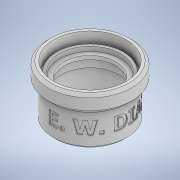
# Autodesk Inventor part: Union_Camara_E_Diaz
Saved by Autodesk Inventor 2021 (Build 250183000, 183)
## iProperties
Created: 2021-02-05
Part Number: Union_Camara_E_Diaz
Material: Generic
Document SubType Name: Modeling
Designer: jorge
Density: 1 g/cm^3
Appearance: Default
Author: jorge
Autodesk Inventor part; units mm, degrees
note: some values were not read from the file. Chosen so that the rebuilt part matches the saved one: direction of "Emboss1".
ref_plane "YZ Plane" through (0, 0, 0) normal (1, 0, 0) x (0, 1, 0)
ref_plane "XZ Plane" through (0, 0, 0) normal (0, 1, 0) x (-1, 0, 0)
ref_plane "XY Plane" through (0, 0, 0) normal (0, 0, 1) x (1, 0, 0)
sketch "Sketch1" plane through (0, 0, 0) normal (0, 1, 0) x (-1, 0, 0)
  circle A0 centre (0, 0) radius 16.8
  circle A1 centre (0, 0) radius 19.8
  dimension "d0" = 33.6
  dimension "d1" = 3
  constraints: 2 centre point, 1 coincident
  measures "d0" diameter of A0
  measures "d1" radial gap between concentric circles of A0 A1
extrude "Extrusion1" add sketch "Sketch1" along normal blind 20
sketch "Sketch2" plane through (0, 20, 0) normal (0, 1, 0) x (1, 0, 0)
  circle A0 centre (0, 0) radius 19.5
  circle A1 centre (0, 0) radius 22.5
  dimension "d4" = 39
  dimension "d5" = 3
  constraints: 2 centre point, 1 coincident
  measures "d4" diameter of A0
  measures "d5" radial gap between concentric circles of A0 A1
extrude "Extrusion2" add sketch "Sketch2" along normal blind 7.5
chamfer "Chamfer1" distance 2.7 angle 45 1 edges at (19.8, 20, 0)
sketch "Sketch3" plane through (0, 20, 0) normal (0, 1, 0) x (1, 0, 0)
  circle A0 centre (0, 0) radius 14
  circle A1 centre (0, 0) radius 16.8
  circle A2 centre (0, 0) radius 16.8 projected
  dimension "d11" = 28
  constraints: 2 centre point, 2 coincident, 1 concentric
  measures "d11" diameter of A0
extrude "Extrusion3" add sketch "Sketch3" against normal blind 2
sketch "Sketch4" plane through (0, 18, 0) normal (0, -1, 0) x (1, 0, 0)
  circle A0 centre (0, 0) radius 15.7
  circle A1 centre (0, 0) radius 16.8
  circle A2 centre (0, 0) radius 16.8 projected
  dimension "d14" = 31.4
  constraints: 2 centre point, 2 coincident, 1 concentric
  measures "d14" diameter of A0
extrude "Extrusion4" add sketch "Sketch4" along normal blind 5
sketch "Sketch5" plane through (0, 27.5, 0) normal (0, 1, 0) x (1, 0, 0)
  circle A0 centre (0, 0) radius 18
  circle A1 centre (0, 0) radius 19.5 projected
  circle A2 centre (0, 0) radius 16.5
  dimension "d17" = 1.5
  dimension "d18" = 3
  constraints: 2 centre point, 2 coincident
  measures "d17" radial gap between concentric circles of A1 A0
  measures "d18" radial gap between concentric circles of A2 A1
extrude "Extrusion5" add sketch "Sketch5" against normal up to surface (7.5 mm away) contours A0
chamfer "Chamfer2" distance 1.5 angle 45 1 edges at (-22.5, 27.5, 0)
sketch "Sketch6" plane through (0, 27.5, 0) normal (0, 1, 0) x (1, 0, 0)
  circle A0 centre (0, 0) radius 18
  circle A1 centre (0, 0) radius 18 projected
  constraints: 1 centre point, 1 coincident, 1 concentric
extrude "Extrusion6" cut sketch "Sketch6" against normal blind 5
chamfer "Chamfer3" distance 1.5 angle 45 1 edges at (19.8, 0, 0)
sketch "Sketch7" plane through (0, 0, 0) normal (1, 0, 0) x (0, 1, 0)
  line L0 (13.6432, 34.118) -> (13.6432, -36.6439) construction
  line L1 (13.6432, -36.6439) -> (5.5986, -36.6439) construction
  line L2 (5.5986, -36.6439) -> (5.5986, 34.118) construction
  line L3 (5.5986, 34.118) -> (13.6432, 34.118) construction
  line L4 (6.6432, 33.3919) -> (13.6432, 33.3919)
  line L5 (13.6432, 33.3919) -> (13.6432, 28.6609)
  line L6 (13.6432, 28.6609) -> (12.3101, 28.6609)
  line L7 (12.3101, 28.6609) -> (12.3101, 31.6447)
  line L8 (12.3101, 31.6447) -> (11.0791, 31.6447)
  line L9 (11.0791, 31.6447) -> (11.0791, 28.8935)
  line L10 (11.0791, 28.8935) -> (9.7461, 28.8935)
  line L11 (9.7461, 28.8935) -> (9.7461, 31.6447)
  line L12 (9.7461, 31.6447) -> (7.9762, 31.6447)
  line L13 (7.9762, 31.6447) -> (7.9762, 28.6609)
  line L14 (7.9762, 28.6609) -> (6.6432, 28.6609)
  line L15 (6.6432, 28.6609) -> (6.6432, 33.3919)
  line L16 (6.6432, 25.8643) -> (6.6432, 27.5264)
  line L17 (6.6432, 27.5264) -> (8.4924, 27.5264)
  line L18 (8.4924, 27.5264) -> (8.4924, 25.8643)
  line L19 (8.4924, 25.8643) -> (6.6432, 25.8643)
  line L20 (13.6432, 12.6188) -> (6.6432, 14.3886)
  line L21 (6.6432, 14.3886) -> (6.6432, 16.3173)
  line L22 (6.6432, 16.3173) -> (10.9714, 17.4405)
  line L23 (10.9714, 17.4405) -> (6.6432, 18.524)
  line L24 (6.6432, 18.524) -> (6.6432, 20.4583)
  line L25 (6.6432, 20.4583) -> (13.6432, 22.2282)
  line L26 (13.6432, 22.2282) -> (13.6432, 20.4016)
  line L27 (13.6432, 20.4016) -> (8.9576, 19.4373)
  line L28 (8.9576, 19.4373) -> (13.6432, 18.2687)
  line L29 (13.6432, 18.2687) -> (13.6432, 16.5216)
  line L30 (13.6432, 16.5216) -> (8.9519, 15.4097)
  line L31 (8.9519, 15.4097) -> (13.6432, 14.4)
  line L32 (13.6432, 14.4) -> (13.6432, 12.6188)
  line L33 (6.6432, 10.1455) -> (6.6432, 11.8076)
  line L34 (6.6432, 11.8076) -> (8.4924, 11.8076)
  line L35 (8.4924, 11.8076) -> (8.4924, 10.1455)
  line L36 (8.4924, 10.1455) -> (6.6432, 10.1455)
  spline S0 degree 2 poles (10.1375, -0.3204) (9.1561, -0.3204) (7.6132, 0.5361) (7.1991, 1.1885) knots 0 0 0 1 2 2 2
  spline S1 degree 2 poles (7.1991, 1.1885) (6.8474, 1.7331) (6.6432, 3.0151) (6.6432, 3.7355) knots 0 0 0 1 2 2 2
  line L37 (6.6432, 3.7355) -> (6.6432, 5.9251)
  line L38 (6.6432, 5.9251) -> (13.6432, 5.9251)
  line L39 (13.6432, 5.9251) -> (13.6432, 3.7582)
  spline S2 degree 2 poles (13.6432, 3.7582) (13.6432, 3.0207) (13.456, 1.7331) (13.0929, 1.1658) knots 0 0 0 1 2 2 2
  spline S3 degree 2 poles (13.0929, 1.1658) (12.6505, 0.4794) (11.1529, -0.3204) (10.1375, -0.3204) knots 0 0 0 1 2 2 2
  spline S4 degree 2 poles (10.1488, 1.4835) (10.8409, 1.4835) (11.8279, 1.96) (12.1059, 2.4478) knots 0 0 0 1 2 2 2
  spline S5 degree 2 poles (12.1059, 2.4478) (12.2988, 2.8052) (12.3385, 3.588) (12.3385, 4.1326) knots 0 0 0 1 2 2 2
  line L40 (12.3385, 4.1326) -> (12.3385, 4.1666)
  line L41 (12.3385, 4.1666) -> (7.9535, 4.1666)
  line L42 (7.9535, 4.1666) -> (7.9535, 4.1326)
  spline S6 degree 2 poles (7.9535, 4.1326) (7.9535, 3.5426) (7.9932, 2.7314) (8.2258, 2.3627) knots 0 0 0 1 2 2 2
  spline S7 degree 2 poles (8.2258, 2.3627) (8.4981, 1.9316) (9.4568, 1.4835) (10.1488, 1.4835) knots 0 0 0 1 2 2 2
  line L43 (6.6432, -4.8472) -> (6.6432, -1.0806)
  line L44 (6.6432, -1.0806) -> (7.8628, -1.0806)
  line L45 (7.8628, -1.0806) -> (7.8628, -2.0846)
  line L46 (7.8628, -2.0846) -> (12.4236, -2.0846)
  line L47 (12.4236, -2.0846) -> (12.4236, -1.0806)
  line L48 (12.4236, -1.0806) -> (13.6432, -1.0806)
  line L49 (13.6432, -1.0806) -> (13.6432, -4.8472)
  line L50 (13.6432, -4.8472) -> (12.4236, -4.8472)
  line L51 (12.4236, -4.8472) -> (12.4236, -3.8431)
  line L52 (12.4236, -3.8431) -> (7.8628, -3.8431)
  line L53 (7.8628, -3.8431) -> (7.8628, -4.8472)
  line L54 (7.8628, -4.8472) -> (6.6432, -4.8472)
  line L55 (6.6432, -5.2613) -> (13.6432, -7.6267)
  line L56 (13.6432, -7.6267) -> (13.6432, -9.5441)
  line L57 (13.6432, -9.5441) -> (6.6432, -11.9096)
  line L58 (6.6432, -11.9096) -> (6.6432, -10.1)
  line L59 (6.6432, -10.1) -> (8.0727, -9.6632)
  line L60 (8.0727, -9.6632) -> (8.0727, -7.4622)
  line L61 (8.0727, -7.4622) -> (6.6432, -7.0198)
  line L62 (6.6432, -7.0198) -> (6.6432, -5.2613)
  line L63 (9.3433, -9.2775) -> (11.6578, -8.5627)
  line L64 (11.6578, -8.5627) -> (9.3433, -7.8423)
  line L65 (9.3433, -7.8423) -> (9.3433, -9.2775)
  line L66 (6.6432, -17.6843) -> (6.6432, -12.1365)
  line L67 (6.6432, -12.1365) -> (7.9535, -12.1365)
  line L68 (7.9535, -12.1365) -> (12.3101, -15.3642)
  line L69 (12.3101, -15.3642) -> (12.3101, -12.3066)
  line L70 (12.3101, -12.3066) -> (13.6432, -12.3066)
  line L71 (13.6432, -12.3066) -> (13.6432, -17.4971)
  line L72 (13.6432, -17.4971) -> (12.3101, -17.4971)
  line L73 (12.3101, -17.4971) -> (7.9762, -14.2807)
  line L74 (7.9762, -14.2807) -> (7.9762, -17.6843)
  line L75 (7.9762, -17.6843) -> (6.6432, -17.6843)
  point P0 (0, 0)
  constraints: 2 other
emboss "Emboss1" sketch "Sketch7" operation cut depth 0.5 direction (-1, 0, 0) wrap yes faces at (-19.7358, 12.0334, -1.5932)
body "Solid1"
